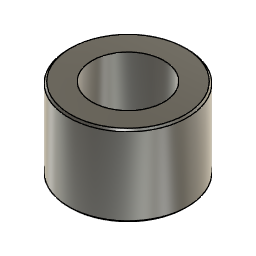
Toebeans v3 (Autodesk Fusion 360 design; units mm, degrees)
Autodesk Fusion 360 part; units mm, degrees
sketch "Sketch1" plane through (0, 0, 0) normal (0, 0, 1) x (1, 0, 0)
  circle A0 centre (0, 0) radius 4
  circle A1 centre (0, 0) radius 6.6
  dimension "d1" = 8
  dimension "d2" = 13.2
  constraint coincident A0.centre A1.centre
  measures "d1" diameter of A0
  measures "d2" diameter of A1
extrude "Extrude1" add sketch "Sketch1" along normal blind 9
chamfer "Chamfer1" distance 0.2 angle 45 1 edges at (-6.1534, -2.3867, 9)
chamfer "Chamfer2" distance 0.2 angle 45 1 edges at (-6.1534, -2.3867, 0)
